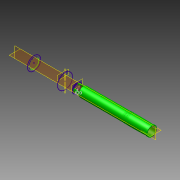
# Autodesk Inventor part: Motor Axle Connector 2
Saved by Autodesk Inventor 2015 (Build 190159000, 159)
## iProperties
Created: 2012-02-20
Part Number: Motor Axle Connector 2
Material: Generic
Document SubType Name: Modeling
Designer: Thom Tremblay
Density: 1 g/cm^3
Appearance: Dark Green
Author: Thom Tremblay
Autodesk Inventor part; units mm, degrees
ref_plane "YZ Plane" through (0, 0, 0) normal (1, 0, 0) x (0, 1, 0)
sketch "Sketch1" plane through (0, 0, 0) normal (0, 0, 1) x (1, 0, 0)
  line L0 (0, 0) -> (1.778, 0)
  line L1 (1.778, 0) -> (1.778, 5.08)
  line L2 (1.778, 5.08) -> (0, 5.08)
  line L3 (0, 5.08) -> (0, 0)
  line L4 (1.778, 0) -> (11.049, 0)
  line L5 (11.049, 0) -> (11.049, 3.683)
  line L6 (11.049, 3.683) -> (1.778, 3.683)
  line L7 (1.778, 3.683) -> (1.778, 0)
  line L8 (8.509, 3.683) -> (6.985, 3.81)
  line L9 (6.985, 3.81) -> (6.985, 3.683)
  line L10 (6.985, 3.683) -> (5.461, 3.81)
  line L11 (5.461, 3.81) -> (5.461, 3.683)
  line L12 (5.461, 3.683) -> (3.937, 3.81)
  line L13 (3.937, 3.81) -> (3.937, 3.683)
  line L14 (0, 0) -> (0, 3.1252)
  line L15 (0, 3.81) -> (0.889, 3.81) construction
  line L16 (0, 3.81) -> (0, 0)
  arc A0 (0, 3.81) -> (-9.906, 3.556) centre (0, -189.484) ccw
  line L17 (-9.906, 3.556) -> (-9.906, 3.81)
  line L18 (-9.906, 3.81) -> (-11.176, 3.81)
  line L19 (-11.176, 3.81) -> (-11.176, 0)
  line L20 (-11.176, 0) -> (0, 0)
  dimension "d0" = 1.778
  dimension "d1" = 10.16
  dimension "d2" = 9.271
  dimension "d3" = 7.366
  dimension "d4" = 7.62
  dimension "d5" = 2.54
  dimension "d6" = 1.524
  dimension "d7" = 7.62
  dimension "d8" = 7.62
  dimension "d9" = 11.176
  dimension "d10" = 7.112
  dimension "d11" = 1.27
  constraints: 42 end point, 8 parallel, 7 perpendicular, 6 point on line, 2 collinear, 2 horizontal, 2 horizontal alignment, 2 point on circle, 1 centre point, 1 tangent
  measures "d0" distance of L1.end L2.end
  measures "d1" diameter of L2 L0
  measures "d2" distance of L5.end L6.end
  measures "d3" diameter of L6 L4
  measures "d4" diameter of L8.end L4
  measures "d5" distance of L5.end L8.start
  measures "d6" horizontal distance of L8.start L8.end
  measures "d7" diameter of L18 L20
  measures "d8" diameter of L15 L20
  measures "d9" distance of L19.end L0.start
  measures "d10" diameter of L17.start L20
  measures "d11" distance of L17.end L18.end
revolve "Revolution1" add sketch "Sketch1" angle 360 about axis through (-11.176, 0, 0) along (1, 0, 0)
sketch "Sketch2" plane through (0, 0, 0) normal (0, 0, 1) x (1, 0, 0)
  line L0 (-11.176, 0.508) -> (-6.096, 0.508)
  line L1 (-6.096, 0.508) -> (-6.096, -0.508)
  line L2 (-6.096, -0.508) -> (-11.176, -0.508)
  line L3 (-11.176, -0.508) -> (-11.176, 0.508)
  line L4 (-11.176, -3.81) -> (-11.176, 3.81) construction
  point P0 (0, 0)
  point P1 (-11.176, 0)
  dimension "d13" = 1.016
  dimension "d14" = 5.08
  constraints: 8 end point, 2 midpoint, 2 parallel, 1 horizontal, 1 perpendicular
  measures "d13" distance of L2.end L0.start
  measures "d14" distance of L0.start L0.end
extrude "Extrusion1" cut sketch "Sketch2" along normal through all both and the other way through all
hole "Hole1" at (-11.176, 0, 0) direction (1, 0, 0) diameter 4.7625 depth 11.1125 counterbore diameter 6.35 counterbore depth 6.35
hole "Hole2" at (11.049, 0, 0) direction (-1, 0, 0) diameter 4.7625 depth 9.525 counterbore diameter 6.35 counterbore depth 1.27
sketch "Sketch3" plane through (1.778, 0, 0) normal (1, 0, 0) x (0, 0, -1)
  circle A0 centre (0, 0) radius 5.08 projected
  circle A1 centre (0, 0) radius 5.08
  circle A2 centre (0, 0) radius 3.683
  circle A3 centre (0, 0) radius 3.81 projected
  circle A4 centre (0, 0) radius 3.81
  circle A5 centre (0, 0) radius 3.81 projected
  circle A6 centre (0, 0) radius 3.683
  constraints: 4 centre point, 4 coincident, 2 concentric
extrude "Extrusion2" cut sketch "Sketch3" against normal blind 1.778 contours A0
extrude "Extrusion3" add sketch "Sketch3" along normal blind 2.159 contours A3
sketch "Sketch4" plane through (11.049, 0, 0) normal (1, 0, 0) x (0, 0, -1)
  circle A0 centre (0, 0) radius 3.683 projected
  circle A1 centre (0, 0) radius 3.175 projected
extrude "Extrusion4" add sketch "Sketch4" along normal blind 29.21
mirror "Mirror1" about plane through (40.259, 0, 0) normal (1, 0, 0) of "Revolution1", "Extrusion1", "Hole1", "Hole2", "Extrusion2", "Extrusion3", "Extrusion4"
ref_plane "Work Plane2" through (25.4, 0, 0) normal (-1, 0, 0) x (0, 0, 1)
sketch "Sketch7" plane through (25.4, 0, 0) normal (-1, 0, 0) x (0, 0, 1)
  circle A0 centre (0, 0) radius 5.715
  line L0 (0, 8.001) -> (0, -8.001) projected
  line L1 (0.635, 6.477) -> (-0.635, 6.477)
  line L2 (-0.635, 6.477) -> (-0.635, 5.6796)
  line L3 (-0.635, 5.461) -> (0, 5.461)
  line L4 (0.635, 5.6796) -> (0.635, 6.477)
  dimension "d43" = 11.43
  dimension "d44" = 0.635
  dimension "d45" = 0.635
  dimension "d46" = 0.254
  dimension "d47" = 0.762
  constraints: 8 end point, 2 parallel, 2 point on circle, 1 centre point, 1 coincident, 1 horizontal, 1 perpendicular, 1 point on line
  measures "d43" diameter of A0
  measures "d44" distance between parallel lines of L0 L2
  measures "d45" distance between parallel lines of L0 L4
  measures "d46" distance edge to line of A0 L3
  measures "d47" distance edge to line of A0 L1
extrude "Extrusion5" add sketch "Sketch7" along normal mid plane 1.27 contours A0 L0 | A0 L0
extrude "Extrusion6" add sketch "Sketch7" along normal mid plane 1.27 contours A0 L0 L1 L4 | A0 L2 L1 L0
pattern_circular "Circular Pattern1" count 13 over 360 about axis through (25.4, 0, 0) along (-1, 0, 0) of "Extrusion6"
ref_plane "Work Plane3" through (34.544, 0, 0) normal (-1, 0, 0) x (0, 0, 1)
sketch "Sketch8" plane through (-11.176, 0, 0) normal (-1, 0, 0) x (0, 0, 1)
  circle A0 centre (0, 0) radius 2.3813 projected
  circle A1 centre (0, 0) radius 16.574
  point P0 (0, 0)
  constraints: 1 centre point, 1 coincident
extrude "Extrusion7" cut sketch "Sketch8" against normal blind 45.72 contours A0 | A1
sketch "Sketch9" plane through (34.544, 0, 0) normal (-1, 0, 0) x (0, 0, 1)
  circle A0 centre (0, 0) radius 3.175 projected
  circle A1 centre (0, 0) radius 3.175
  circle A2 centre (0, 0) radius 2.667
  circle A3 centre (0, 0) radius 3.683 projected
  circle A4 centre (0, 0) radius 3.683
  dimension "d58" = 0.508
  constraints: 3 centre point, 3 coincident, 2 concentric
  measures "d58" radial gap between concentric circles of A0 A2
extrude "Extrusion8" add sketch "Sketch9" against normal blind 10.16 contours A0
extrude "Extrusion9" cut sketch "Sketch9" against normal blind 5.08 contours A3
sketch "Sketch10" plane through (0, 0, 0) normal (0, 0, 1) x (1, 0, 0)
  line L0 (34.544, -2.667) -> (44.704, -2.667) projected
  line L1 (34.544, -3.175) -> (39.624, -3.175) projected
  line L2 (-18.3388, 0) -> (110.0328, 0) projected
  line L3 (34.544, 3.175) -> (39.624, 3.175)
  line L4 (39.624, 3.175) -> (39.624, 2.667)
  line L5 (39.624, 2.667) -> (34.544, 2.667)
  line L6 (34.544, 2.667) -> (34.544, 3.175)
  line L7 (34.544, -3.175) -> (39.624, -3.175)
  line L8 (39.624, -3.175) -> (39.624, -2.667)
  line L9 (39.624, -2.667) -> (34.544, -2.667)
  line L10 (34.544, -2.667) -> (34.544, -3.175)
  point P0 (0, 0)
  dimension "d63" = 5.08
  constraints: 16 end point, 2 parallel, 2 symmetric about line, 1 horizontal, 1 perpendicular
  measures "d63" distance of L4.end L5.end
revolve "Revolution2" cut sketch "Sketch10" angle 65 about axis through (0, 0, 0) along (1, 0, 0)
sketch "Sketch11" plane through (0, 0, 0) normal (0, 0, 1) x (1, 0, 0)
  line L0 (39.624, 3.175) -> (37.084, 3.175)
  line L1 (37.084, 3.175) -> (37.084, 2.667)
  line L2 (37.084, 2.667) -> (39.624, 2.667)
  line L3 (39.624, 2.667) -> (39.624, 3.175)
  line L4 (34.544, 1.1271) -> (39.624, 1.1271) projected
  line L5 (-18.3388, 0) -> (110.0328, 0) projected
  line L6 (39.624, -3.175) -> (37.084, -3.175)
  line L7 (37.084, -3.175) -> (37.084, -2.667)
  line L8 (37.084, -2.667) -> (39.624, -2.667)
  line L9 (39.624, -2.667) -> (39.624, -3.175)
  point P0 (0, 0)
  dimension "d65" = 2.54
  constraints: 16 end point, 4 symmetric about line, 2 parallel, 1 horizontal, 1 perpendicular
  measures "d65" distance of L2.end L1.end
revolve "Revolution3" cut sketch "Sketch11" angle 30 about axis through (0, 0, 0) along (-1, 0, 0)
sketch "Sketch12" plane through (37.084, 2.667, 0) normal (1, 0, 0) x (0, 0, -1)
  line L0 (1.3335, -0.3573) -> (1.5875, 0.0826) projected
  line L1 (-1.3335, -4.9767) -> (-1.5875, -5.4166) projected
  arc A0 (2.8775, -4.0088) -> (0, 0.508) centre (0, -2.667) ccw projected
  arc A1 (2.4171, -3.7941) -> (0, 0) centre (0, -2.667) ccw projected
  line L2 (0, 0) -> (0, 0.508) projected
  arc A2 (-2.4171, -1.5399) -> (0, -5.334) centre (0, -2.667) ccw projected
  arc A3 (-2.8775, -1.3252) -> (0, -5.842) centre (0, -2.667) ccw projected
  line L3 (0, -5.334) -> (0, -5.842) projected
  arc A4 (1.5875, 0.0826) -> (1.4695, 0.1475) centre (0, -2.667) ccw
  arc A5 (1.3335, -0.3573) -> (1.2152, -0.2929) centre (0, -2.667) ccw
  line L4 (1.3335, -0.3573) -> (1.5875, 0.0826)
  line L5 (1.2152, -0.2929) -> (1.4695, 0.1475)
  arc A6 (-1.5875, -5.4166) -> (-1.4695, -5.4815) centre (0, -2.667) ccw
  arc A7 (-1.3335, -4.9767) -> (-1.2152, -5.0411) centre (0, -2.667) ccw
  line L6 (-1.3335, -4.9767) -> (-1.5875, -5.4166)
  line L7 (-1.4695, -5.4815) -> (-1.2152, -5.0411)
  dimension "d67" = 0.1346
  dimension "d68" = 0.1346
  constraints: 11 point on circle, 8 end point, 4 centre point, 4 concentric, 2 collinear, 2 parallel
  measures "d67" distance between parallel lines of L0 L5
  measures "d68" distance between parallel lines of L7 L1
extrude "Extrusion10" cut sketch "Sketch12" against normal blind 0.1346 contours A1 L5 A0 L0 | A2 L7 A3 L1
chamfer "Chamfer1" distance 0.1346 angle 45 2 edges at (36.9494, 2.5297, -1.4605) (36.9494, -2.5297, 1.4605)
equation "\"d8\" = d7"
body "Solid1"
